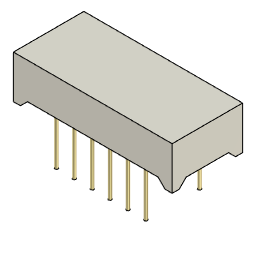
3 digit 7 segment display v3 (Autodesk Fusion 360 design; units mm, degrees)
Autodesk Fusion 360 part; units mm, degrees
note: some values were not read from the file. Set by a fixed rule: which face or edge a step refers to.
sketch "Sketch1" plane through (0, 0, 0) normal (0, 0, 1) x (1, 0, 0)
  line L0 (11.265, -5) -> (-11.265, -5)
  line L1 (-11.265, -5) -> (-11.265, 5)
  line L2 (-11.265, 5) -> (11.265, 5)
  line L3 (11.265, 5) -> (11.265, -5)
  line L4 (11.265, -5) -> (-11.265, 5) construction
  line L5 (-11.265, -5) -> (11.265, 5) construction
  line L6 (-11.265, 0) -> (11.265, 0)
  line L7 (0, 5) -> (0, -5)
  circle A0 centre (-6.35, 3.81) radius 0.225
  circle A1 centre (-3.81, 3.81) radius 0.225
  circle A2 centre (-1.27, 3.81) radius 0.225
  circle A3 centre (1.27, 3.81) radius 0.225
  circle A4 centre (3.81, 3.81) radius 0.225
  circle A5 centre (6.35, 3.81) radius 0.225
  circle A6 centre (-6.35, -3.81) radius 0.225
  circle A7 centre (-3.81, -3.81) radius 0.225
  circle A8 centre (-1.27, -3.81) radius 0.225
  circle A9 centre (1.27, -3.81) radius 0.225
  circle A10 centre (3.81, -3.81) radius 0.225
  circle A11 centre (6.35, -3.81) radius 0.225
  dimension "d1" = 22.53
  dimension "d2" = 10
  dimension "d4" = 0.45
  dimension "d5" = 12.7
  dimension "d6" = 7.62
  dimension "d9" = 2.54
  dimension "d10" = -7.62
  constraint horizontal L0
  constraint perpendicular L0 L1
  constraint parallel L0 L2
  constraint parallel L1 L3
  constraint coincident L4 origin
  constraint coincident L5 origin
  constraint midpoint L1 L6.start
  constraint midpoint L3 L6.end
  constraint midpoint L2 L7.start
  constraint midpoint L0 L7.end
  measures "d1" distance of L1.end L2.end
  measures "d2" distance of L0.start L2.end
  measures "d4" diameter of A0
extrude "Extrude1" add sketch "Sketch1" along normal blind 6.1 contours L0 L3 L6 L7 | L0 L1 L6 L7 | L2 L3 L6 L7 | L1 L2 L6 L7 | A0 | A1 | A2 | A3 | A4 | A5 | A6 | A7 | A8 | A9 | A10 | A11
sketch "Sketch2" plane through (0, -5, 0) normal (0, -1, 0) x (1, 0, 0)
  line L0 (-11.265, 0) -> (11.265, 0)
  line L1 (11.265, 0) -> (11.265, 6.1)
  line L2 (11.265, 6.1) -> (-11.265, 6.1)
  line L3 (-11.265, 6.1) -> (-11.265, 0)
  line L4 (-10.265, 0) -> (-9.265, 1)
  line L5 (-9.265, 1) -> (9.265, 1)
  line L6 (9.265, 1) -> (10.265, 0)
  line L7 (11.265, 0) -> (-11.265, 0)
  line L8 (0, 0) -> (0, 6.1)
  point P0 (-11.265, 0)
  point P1 (11.265, 0)
  dimension "d15" = 1
  dimension "d16" = 1
  dimension "d17" = 1
  dimension "d26" = 45
  constraint coincident L0 L4.start
  constraint parallel L0 L5
  constraint coincident L0 L6.end
  constraint coincident L8.start origin
  constraint midpoint L2 L8.end
  constraint symmetric L4 L6 L8
  measures "d15" distance of L4.start P0
  measures "d16" distance of L6.end P1
  measures "d17" distance of L5 L7
  measures "d26" angle of L4 L7
extrude "Extrude3" cut sketch "Sketch2" against normal up to surface (10 mm away) contours L0 L4 L5 L7 L8 | L0 L5 L6 L7 L8
sketch "Sketch3" plane through (-11.265, 0, 0) normal (-1, 0, 0) x (0, -1, 0)
  line L0 (-5, 0) -> (5, 0)
  line L1 (5, 0) -> (5, 6.1)
  line L2 (5, 6.1) -> (-5, 6.1)
  line L3 (-5, 6.1) -> (-5, 0)
  line L4 (-4, 0) -> (-3, 1)
  line L5 (-3, 1) -> (3, 1)
  line L6 (3, 1) -> (4, 0)
  line L7 (5, 0) -> (-5, 0)
  line L8 (-5, 0) -> (-4, 0)
  line L9 (0, 0) -> (0, 6.1)
  dimension "d22" = 1
  dimension "d23" = 1
  dimension "d24" = 1
  dimension "d25" = 45
  constraint coincident L0 L4.start
  constraint parallel L0 L5
  constraint coincident L0 L6.end
  constraint coincident L0.start L3.end
  constraint coincident L9.start origin
  constraint midpoint L2 L9.end
  constraint symmetric L4 L6 L9
  measures "d22" distance of L5 L7
  measures "d23" distance of L1 L6.end
  measures "d24" distance of L4.start L0.start
  measures "d25" angle of L4 L7
extrude "Extrude4" cut sketch "Sketch3" against normal up to surface (22.53 mm away) contours L0 L4 L5 L7 L9 | L0 L5 L6 L7 L9
extrude "Extrude2" add sketch "Sketch1" against normal blind 7.3 from surface at 1 contours A0 | A1 | A2 | A3 | A4 | A5 | A6 | A7 | A8 | A9 | A10 | A11
equation "d5 = ( 2.54 * 5 ) * 1 mm"
equation "d13 = -6.30 mm - 1 mm"
